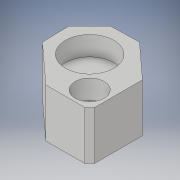
# Autodesk Inventor part: test_fit_3_5
Saved by Autodesk Inventor 2019 (Build 230136000, 136)
## iProperties
Created: 2019-04-10
Part Number: test_fit_3_5
Material: Generic
Document SubType Name: Modeling
Designer: jmc
Density: 1 g/cm^3
Appearance: Default
Author: jmc
## iProperties of the stored document test_fit_3_5_3DPrint.ipt
Created: 2019-04-10
Part Number: test_fit_3_5_3DPrint
Material: Generic
Document SubType Name: Modeling
Designer: jmc
Density: 1 g/cm^3
Appearance: Default
Author: jmc
Autodesk Inventor part; units mm, degrees
ref_plane "YZ Plane" through (0, 0, 0) normal (1, 0, 0) x (0, 1, 0)
ref_plane "XZ Plane" through (0, 0, 0) normal (0, 1, 0) x (-1, 0, 0)
ref_plane "XY Plane" through (0, 0, 0) normal (0, 0, 1) x (1, 0, 0)
sketch "Sketch1" plane through (0, 0, 0) normal (0, 1, 0) x (-1, 0, 0)
  line L0 (-0.4846, 5) -> (-5, 5)
  line L1 (-5, 5) -> (-5, -0.4418)
  line L2 (2.3844, 2.3844) -> (-2.6156, -2.6156) construction
  line L3 (-5, 5) -> (2.5, -2.5) construction
  circle A0 centre (0, 0) radius 2.5
  circle A1 centre (-3.1787, 3.1787) radius 1.5
  line L4 (-0.4846, 5) -> (5, 0)
  line L5 (5, 0) -> (0, -5)
  line L6 (0, -5) -> (-5, -0.4418)
  dimension "d2" = 5
  dimension "d3" = 3
  constraints: 14 end point, 5 point on line, 2 centre point, 1 coincident, 1 horizontal, 1 midpoint, 1 parallel, 1 perpendicular
  measures "d2" diameter of A0
  measures "d3" diameter of A1
extrude "Extrusion1" add sketch "Sketch1" along normal blind 5
sketch "Sketch2" plane through (0, 0, 0) normal (0, -1, 0) x (1, 0, 0)
  circle A0 centre (0, 0) radius 2.5 projected
  circle A1 centre (3.1787, 3.1787) radius 1.5 projected
extrude "Extrusion2" add sketch "Sketch2" against normal blind 3
chamfer "Chamfer1" distance 2 angle 45 2 edges at (0, 2.5, -5) (-5, 2.5, 0)
chamfer "Chamfer2" distance 0.5 angle 45 1 edges at (5, 2.5, 5)
body "Solid1"
